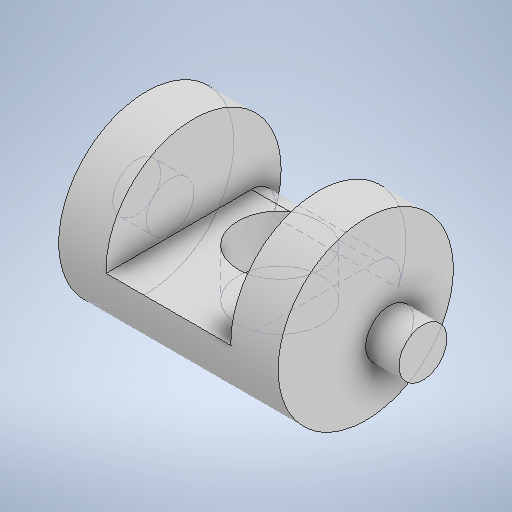
# Autodesk Inventor part: custom_cam
Saved by Autodesk Inventor 2025.1 (Build 291241000, 241)
## iProperties
Created: 2025-07-23
Part Number: custom_cam
Material: Generic
Document SubType Name: Modeling
Designer: santiago
Density: 1 g/cm^3
Appearance: Default
Author: santiago
Autodesk Inventor part; units mm, degrees
ref_plane "YZ Plane" through (0, 0, 0) normal (1, 0, 0) x (0, 1, 0)
ref_plane "XZ Plane" through (0, 0, 0) normal (0, 1, 0) x (-1, 0, 0)
ref_plane "XY Plane" through (0, 0, 0) normal (0, 0, 1) x (1, 0, 0)
sketch "Sketch1" plane through (0, 0, 0) normal (1, 0, 0) x (0, 1, 0)
  circle A0 centre (0, 0) radius 1.5
  dimension "d0" = 3
  constraints: 1 centre point, 1 coincident
  measures "d0" diameter of A0
extrude "Extrusion1" add sketch "Sketch1" along normal mid plane 18
sketch "Sketch2" plane through (0, 0, 0) normal (1, 0, 0) x (0, 1, 0)
  circle A0 centre (1.5, 1.5) radius 5.5
  point P0 (0, 0)
  dimension "cam_size" = 11
  dimension "top_ex" = 1.5
  dimension "d14" = 1.5
  constraints: 1 centre point
  measures "cam_size" diameter of A0
  measures "top_ex" horizontal distance of point (0, 0) A0.centre
  measures "d14" horizontal distance of point (0, 0) A0.centre
extrude "Extrusion2" add sketch "Sketch2" along normal mid plane 13.8
sketch "Sketch3" plane through (0, 0, 0) normal (1, 0, 0) x (0, 1, 0)
  circle A0 centre (1.5, 1.5) radius 5.5 projected
  line L0 (1.3393, 6.9977) -> (1.3393, -3.5197)
  circle A1 centre (-0.1607, -2.139) radius 1.5
  point P0 (0, 0)
  point P1 (1.3393, -2.139)
  point P2 (-0.7835, -3.5036)
  dimension "d8" = 3
  constraints: 2 end point, 1 centre point, 1 tangent, 1 vertical, 3 other
  measures "d8" diameter of A1
extrude "Extrusion3" cut sketch "Sketch3" along normal mid plane 7.85 contours A0 A1 L0 picked at (1.7559, 3.9166)
sketch "Sketch4" plane through (-3.925, 1.3393, -2.139) normal (0, 1, 0) x (1, 0, 0)
  circle A0 centre (3.925, -2.139) radius 2.625
  line L0 (-5.075, -0.639) -> (-5.075, -3.639) projected
  point P0 (-5.075, -2.139)
  dimension "d11" = 5.25
  constraints: 1 centre point, 1 coincident, 1 horizontal alignment, 1 midpoint
  measures "d11" diameter of A0
extrude "Extrusion4" cut sketch "Sketch4" against normal blind 3
body "Solid1"
